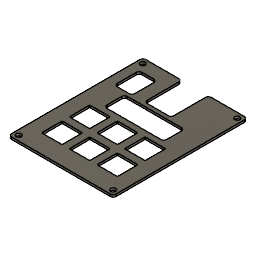
JONAHS LID (Autodesk Fusion 360 design; units mm, degrees)
part number: 2026-01-23-16-47-23-754
Autodesk Fusion 360 part; units mm, degrees
note: some values were not read from the file. Chosen so that the rebuilt part matches the saved one: which face or edge a step refers to; which pieces of a blend or face edit are solid. Set by a fixed rule: which sketch regions a step uses.
sketch "Sketch3" plane through (0, 0, 1.51) normal (0, 0, 1) x (-1, 0, 0)
  line L0 (-26.1938, 109.5375) -> (-88.1063, 109.5375)
  line L1 (-88.1063, 109.5375) -> (-88.1063, 27.245)
  line L2 (-88.1063, 27.245) -> (-26.1938, 27.245)
  line L3 (-26.1937, 27.245) -> (-26.1938, 109.5375)
  circle A0 centre (-33.02, 95.25) radius 0.85
  circle A1 centre (-34.29, 92.71) radius 0.75
  circle A2 centre (-38.1, 95.25) radius 2
  arc A3 (-43.3613, 96.0804) -> (-42.6772, 94.5646) centre (-43.18, 95.25) ccw
  arc A4 (-42.6772, 94.5646) -> (-43.3613, 96.0804) centre (-43.18, 95.25) ccw
  arc A5 (-40.9927, 90.8319) -> (-40.377, 89.4676) centre (-40.64, 90.17) ccw
  arc A6 (-40.377, 89.4676) -> (-40.9927, 90.8319) centre (-40.64, 90.17) ccw
  line L4 (-45.8755, 103.7524) -> (-46.5158, 103.0702)
  line L5 (-46.5158, 103.0702) -> (-46.5783, 103.1039)
  line L6 (-46.5783, 103.1039) -> (-46.8305, 103.1722)
  line L7 (-46.8305, 103.1722) -> (-48.4195, 103.1722)
  line L8 (-48.4195, 103.1722) -> (-48.6135, 103.1355)
  line L9 (-48.6135, 103.1355) -> (-48.6717, 103.1039)
  line L10 (-48.6717, 103.1039) -> (-49.403, 103.6875)
  line L11 (-49.403, 103.6875) -> (-49.3745, 103.7524)
  line L12 (-49.3745, 103.7524) -> (-49.325, 103.9693)
  line L13 (-49.325, 103.9693) -> (-49.325, 105.375)
  line L14 (-49.325, 105.375) -> (-49.3515, 105.5406)
  line L15 (-49.3515, 105.5406) -> (-49.3745, 105.5919)
  line L16 (-49.3745, 105.5919) -> (-48.7342, 106.2741)
  line L17 (-48.7342, 106.2741) -> (-48.6717, 106.2405)
  line L18 (-48.6717, 106.2405) -> (-48.4195, 106.1722)
  line L19 (-48.4195, 106.1722) -> (-46.8305, 106.1722)
  line L20 (-46.8305, 106.1722) -> (-46.6365, 106.2088)
  line L21 (-46.6365, 106.2088) -> (-46.5783, 106.2405)
  line L22 (-46.5783, 106.2405) -> (-45.847, 105.6568)
  line L23 (-45.847, 105.6568) -> (-45.8755, 105.5919)
  line L24 (-45.8755, 105.5919) -> (-45.925, 105.375)
  line L25 (-45.925, 105.375) -> (-45.925, 103.9693)
  line L26 (-45.925, 103.9693) -> (-45.8985, 103.8037)
  line L27 (-45.8985, 103.8037) -> (-45.8755, 103.7524)
  circle A7 centre (-52.07, 95.25) radius 0.85
  circle A8 centre (-53.34, 92.71) radius 0.75
  circle A9 centre (-57.15, 95.25) radius 2
  circle A10 centre (-33.02, 76.2) radius 0.85
  circle A11 centre (-34.29, 73.66) radius 0.75
  circle A12 centre (-38.1, 76.2) radius 2
  circle A13 centre (-43.18, 76.2) radius 0.85
  circle A14 centre (-40.64, 71.12) radius 0.75
  line L28 (-45.8105, 84.7036) -> (-46.4508, 84.0214)
  line L29 (-46.4508, 84.0214) -> (-46.5133, 84.0551)
  line L30 (-46.5133, 84.0551) -> (-46.7655, 84.1234)
  line L31 (-46.7655, 84.1234) -> (-48.3545, 84.1234)
  line L32 (-48.3545, 84.1234) -> (-48.5485, 84.0867)
  line L33 (-48.5485, 84.0867) -> (-48.6067, 84.0551)
  line L34 (-48.6067, 84.0551) -> (-49.338, 84.6387)
  line L35 (-49.338, 84.6387) -> (-49.3095, 84.7036)
  line L36 (-49.3095, 84.7036) -> (-49.26, 84.9205)
  line L37 (-49.26, 84.9205) -> (-49.26, 86.3262)
  line L38 (-49.26, 86.3262) -> (-49.2865, 86.4918)
  line L39 (-49.2865, 86.4918) -> (-49.3095, 86.5431)
  line L40 (-49.3095, 86.5431) -> (-48.6692, 87.2253)
  line L41 (-48.6692, 87.2253) -> (-48.6067, 87.1917)
  line L42 (-48.6067, 87.1917) -> (-48.3545, 87.1234)
  line L43 (-48.3545, 87.1234) -> (-46.7655, 87.1234)
  line L44 (-46.7655, 87.1234) -> (-46.5715, 87.16)
  line L45 (-46.5715, 87.16) -> (-46.5133, 87.1917)
  line L46 (-46.5133, 87.1917) -> (-45.782, 86.608)
  line L47 (-45.782, 86.608) -> (-45.8105, 86.5431)
  line L48 (-45.8105, 86.5431) -> (-45.86, 86.3262)
  line L49 (-45.86, 86.3262) -> (-45.86, 84.9205)
  line L50 (-45.86, 84.9205) -> (-45.8335, 84.7549)
  line L51 (-45.8335, 84.7549) -> (-45.8105, 84.7036)
  circle A15 centre (-52.07, 76.2) radius 0.85
  circle A16 centre (-53.34, 73.66) radius 0.75
  arc A17 (-59.1453, 76.3366) -> (-57.5161, 74.2338) centre (-57.15, 76.2) ccw
  arc A18 (-57.5161, 74.2338) -> (-59.1453, 76.3366) centre (-57.15, 76.2) ccw
  line L52 (-64.9255, 103.7524) -> (-65.5658, 103.0702)
  line L53 (-65.5658, 103.0702) -> (-65.6283, 103.1039)
  line L54 (-65.6283, 103.1039) -> (-65.8805, 103.1722)
  line L55 (-65.8805, 103.1722) -> (-67.4695, 103.1722)
  line L56 (-67.4695, 103.1722) -> (-67.6635, 103.1355)
  line L57 (-67.6635, 103.1355) -> (-67.7217, 103.1039)
  line L58 (-67.7217, 103.1039) -> (-68.453, 103.6875)
  line L59 (-68.453, 103.6875) -> (-68.4245, 103.7524)
  line L60 (-68.4245, 103.7524) -> (-68.375, 103.9693)
  line L61 (-68.375, 103.9693) -> (-68.375, 105.375)
  line L62 (-68.375, 105.375) -> (-68.4015, 105.5406)
  line L63 (-68.4015, 105.5406) -> (-68.4245, 105.5919)
  line L64 (-68.4245, 105.5919) -> (-67.7842, 106.2741)
  line L65 (-67.7842, 106.2741) -> (-67.7217, 106.2405)
  line L66 (-67.7217, 106.2405) -> (-67.4695, 106.1722)
  line L67 (-67.4695, 106.1722) -> (-65.8805, 106.1722)
  line L68 (-65.8805, 106.1722) -> (-65.6865, 106.2088)
  line L69 (-65.6865, 106.2088) -> (-65.6283, 106.2405)
  line L70 (-65.6283, 106.2405) -> (-64.897, 105.6568)
  line L71 (-64.897, 105.6568) -> (-64.9255, 105.5919)
  line L72 (-64.9255, 105.5919) -> (-64.975, 105.375)
  line L73 (-64.975, 105.375) -> (-64.975, 103.9693)
  line L74 (-64.975, 103.9693) -> (-64.9485, 103.8037)
  line L75 (-64.9485, 103.8037) -> (-64.9255, 103.7524)
  circle A19 centre (-62.23, 95.25) radius 0.85
  circle A20 centre (-59.69, 90.17) radius 0.75
  circle A21 centre (-71.12, 95.25) radius 0.85
  circle A22 centre (-72.39, 92.71) radius 0.75
  circle A23 centre (-76.2, 95.25) radius 2
  circle A24 centre (-81.28, 95.25) radius 0.85
  circle A25 centre (-78.74, 90.17) radius 0.75
  line L76 (-64.4728, 84.7212) -> (-65.1131, 84.039)
  line L77 (-65.1131, 84.039) -> (-65.1756, 84.0727)
  line L78 (-65.1756, 84.0727) -> (-65.4278, 84.141)
  line L79 (-65.4278, 84.141) -> (-67.0168, 84.141)
  line L80 (-67.0168, 84.141) -> (-67.2108, 84.1043)
  line L81 (-67.2108, 84.1043) -> (-67.269, 84.0727)
  line L82 (-67.269, 84.0727) -> (-68.0003, 84.6563)
  line L83 (-68.0003, 84.6563) -> (-67.9718, 84.7212)
  line L84 (-67.9718, 84.7212) -> (-67.9223, 84.9381)
  line L85 (-67.9223, 84.9381) -> (-67.9223, 86.3438)
  line L86 (-67.9223, 86.3438) -> (-67.9488, 86.5094)
  line L87 (-67.9488, 86.5094) -> (-67.9718, 86.5607)
  line L88 (-67.9718, 86.5607) -> (-67.3315, 87.2429)
  line L89 (-67.3315, 87.2429) -> (-67.269, 87.2093)
  line L90 (-67.269, 87.2093) -> (-67.0168, 87.141)
  line L91 (-67.0168, 87.141) -> (-65.4278, 87.141)
  line L92 (-65.4278, 87.141) -> (-65.2338, 87.1776)
  line L93 (-65.2338, 87.1776) -> (-65.1756, 87.2093)
  line L94 (-65.1756, 87.2093) -> (-64.4443, 86.6256)
  line L95 (-64.4443, 86.6256) -> (-64.4728, 86.5607)
  line L96 (-64.4728, 86.5607) -> (-64.5223, 86.3438)
  line L97 (-64.5223, 86.3438) -> (-64.5223, 84.9381)
  line L98 (-64.5223, 84.9381) -> (-64.4958, 84.7725)
  line L99 (-64.4958, 84.7725) -> (-64.4728, 84.7212)
  circle A26 centre (-68.95, 78.7) radius 0.5
  circle A27 centre (-62.23, 76.2) radius 0.85
  circle A28 centre (-59.69, 71.12) radius 0.75
  circle A29 centre (-68.95, 76.2) radius 0.5
  circle A30 centre (-68.95, 73.7) radius 0.5
  arc A31 (-77.1, 82.55) -> (-77.1, 81.05) centre (-77.1, 81.8) ccw
  line L100 (-77.1, 82.55) -> (-75.8, 82.55)
  arc A32 (-75.8, 81.05) -> (-75.8, 82.55) centre (-75.8, 81.8) ccw
  line L101 (-75.8, 81.05) -> (-77.1, 81.05)
  circle A33 centre (-83.45, 78.7) radius 0.5
  arc A34 (-77.1, 71.35) -> (-77.1, 69.85) centre (-77.1, 70.6) ccw
  line L102 (-77.1, 71.35) -> (-75.8, 71.35)
  arc A35 (-75.8, 69.85) -> (-75.8, 71.35) centre (-75.8, 70.6) ccw
  line L103 (-75.8, 69.85) -> (-77.1, 69.85)
  circle A36 centre (-83.45, 73.7) radius 0.5
  circle A37 centre (-40.4813, 61.9125) radius 0.5
  circle A38 centre (-40.4813, 59.3725) radius 0.5
  line L104 (-31.588, 56.1274) -> (-32.2283, 55.4452)
  line L105 (-32.2283, 55.4452) -> (-32.2908, 55.4789)
  line L106 (-32.2908, 55.4789) -> (-32.543, 55.5472)
  line L107 (-32.543, 55.5472) -> (-34.132, 55.5472)
  line L108 (-34.132, 55.5472) -> (-34.326, 55.5105)
  line L109 (-34.326, 55.5105) -> (-34.3842, 55.4789)
  line L110 (-34.3842, 55.4789) -> (-35.1155, 56.0625)
  line L111 (-35.1155, 56.0625) -> (-35.087, 56.1274)
  line L112 (-35.087, 56.1274) -> (-35.0375, 56.3443)
  line L113 (-35.0375, 56.3443) -> (-35.0375, 57.75)
  line L114 (-35.0375, 57.75) -> (-35.064, 57.9156)
  line L115 (-35.064, 57.9156) -> (-35.087, 57.9669)
  line L116 (-35.087, 57.9669) -> (-34.4467, 58.6491)
  line L117 (-34.4467, 58.6491) -> (-34.3842, 58.6155)
  line L118 (-34.3842, 58.6155) -> (-34.132, 58.5472)
  line L119 (-34.132, 58.5472) -> (-32.543, 58.5472)
  line L120 (-32.543, 58.5472) -> (-32.349, 58.5838)
  line L121 (-32.349, 58.5838) -> (-32.2908, 58.6155)
  line L122 (-32.2908, 58.6155) -> (-31.5595, 58.0318)
  line L123 (-31.5595, 58.0318) -> (-31.588, 57.9669)
  line L124 (-31.588, 57.9669) -> (-31.6375, 57.75)
  line L125 (-31.6375, 57.75) -> (-31.6375, 56.3443)
  line L126 (-31.6375, 56.3443) -> (-31.611, 56.1787)
  line L127 (-31.611, 56.1787) -> (-31.588, 56.1274)
  arc A39 (-40.8929, 57.1164) -> (-40.3451, 56.3514) centre (-40.4813, 56.8325) ccw
  arc A40 (-40.3451, 56.3514) -> (-40.8929, 57.1164) centre (-40.4813, 56.8325) ccw
  circle A41 centre (-40.4813, 54.2925) radius 0.5
  line L128 (-45.8755, 65.6524) -> (-46.5158, 64.9702)
  line L129 (-46.5158, 64.9702) -> (-46.5783, 65.0039)
  line L130 (-46.5783, 65.0039) -> (-46.8305, 65.0722)
  line L131 (-46.8305, 65.0722) -> (-48.4195, 65.0722)
  line L132 (-48.4195, 65.0722) -> (-48.6135, 65.0355)
  line L133 (-48.6135, 65.0355) -> (-48.6717, 65.0039)
  line L134 (-48.6717, 65.0039) -> (-49.403, 65.5875)
  line L135 (-49.403, 65.5875) -> (-49.3745, 65.6524)
  line L136 (-49.3745, 65.6524) -> (-49.325, 65.8693)
  line L137 (-49.325, 65.8693) -> (-49.325, 67.275)
  line L138 (-49.325, 67.275) -> (-49.3515, 67.4406)
  line L139 (-49.3515, 67.4406) -> (-49.3745, 67.4919)
  line L140 (-49.3745, 67.4919) -> (-48.7342, 68.1741)
  line L141 (-48.7342, 68.1741) -> (-48.6717, 68.1405)
  line L142 (-48.6717, 68.1405) -> (-48.4195, 68.0722)
  line L143 (-48.4195, 68.0722) -> (-46.8305, 68.0722)
  line L144 (-46.8305, 68.0722) -> (-46.6365, 68.1088)
  line L145 (-46.6365, 68.1088) -> (-46.5783, 68.1405)
  line L146 (-46.5783, 68.1405) -> (-45.847, 67.5568)
  line L147 (-45.847, 67.5568) -> (-45.8755, 67.4919)
  line L148 (-45.8755, 67.4919) -> (-45.925, 67.275)
  line L149 (-45.925, 67.275) -> (-45.925, 65.8693)
  line L150 (-45.925, 65.8693) -> (-45.8985, 65.7037)
  line L151 (-45.8985, 65.7037) -> (-45.8755, 65.6524)
  line L152 (-55.6192, 57.8615) -> (-56.2595, 57.1793)
  line L153 (-56.2595, 57.1793) -> (-56.322, 57.213)
  line L154 (-56.322, 57.213) -> (-56.5742, 57.2813)
  line L155 (-56.5742, 57.2813) -> (-58.1632, 57.2813)
  line L156 (-58.1632, 57.2813) -> (-58.3572, 57.2446)
  line L157 (-58.3572, 57.2446) -> (-58.4154, 57.213)
  line L158 (-58.4154, 57.213) -> (-59.1467, 57.7966)
  line L159 (-59.1467, 57.7966) -> (-59.1182, 57.8615)
  line L160 (-59.1182, 57.8615) -> (-59.0687, 58.0784)
  line L161 (-59.0687, 58.0784) -> (-59.0687, 59.4841)
  line L162 (-59.0687, 59.4841) -> (-59.0952, 59.6497)
  line L163 (-59.0952, 59.6497) -> (-59.1182, 59.701)
  line L164 (-59.1182, 59.701) -> (-58.4779, 60.3832)
  line L165 (-58.4779, 60.3832) -> (-58.4154, 60.3496)
  line L166 (-58.4154, 60.3496) -> (-58.1632, 60.2813)
  line L167 (-58.1632, 60.2813) -> (-56.5742, 60.2813)
  line L168 (-56.5742, 60.2813) -> (-56.3802, 60.3179)
  line L169 (-56.3802, 60.3179) -> (-56.322, 60.3496)
  line L170 (-56.322, 60.3496) -> (-55.5907, 59.7659)
  line L171 (-55.5907, 59.7659) -> (-55.6192, 59.701)
  line L172 (-55.6192, 59.701) -> (-55.6687, 59.4841)
  line L173 (-55.6687, 59.4841) -> (-55.6687, 58.0784)
  line L174 (-55.6687, 58.0784) -> (-55.6422, 57.9128)
  line L175 (-55.6422, 57.9128) -> (-55.6192, 57.8615)
  line L176 (-43.4606, 36.3505) -> (-43.8063, 36.3152)
  line L177 (-43.8063, 36.3152) -> (-43.9369, 36.3706)
  line L178 (-43.9369, 36.3706) -> (-44.1428, 36.9908)
  line L179 (-44.1428, 36.9908) -> (-44.1092, 37.0533)
  line L180 (-44.1092, 37.0533) -> (-44.0409, 37.3055)
  line L181 (-44.0409, 37.3055) -> (-44.0409, 38.8945)
  line L182 (-44.0409, 38.8945) -> (-44.0775, 39.0885)
  line L183 (-44.0775, 39.0885) -> (-44.1092, 39.1467)
  line L184 (-44.1092, 39.1467) -> (-43.5255, 39.878)
  line L185 (-43.5255, 39.878) -> (-43.4606, 39.8495)
  line L186 (-43.4606, 39.8495) -> (-43.2437, 39.8)
  line L187 (-43.2437, 39.8) -> (-41.838, 39.8)
  line L188 (-41.838, 39.8) -> (-41.6724, 39.8265)
  line L189 (-41.6724, 39.8265) -> (-41.6211, 39.8495)
  line L190 (-41.6211, 39.8495) -> (-40.9389, 39.2092)
  line L191 (-40.9389, 39.2092) -> (-40.9726, 39.1467)
  line L192 (-40.9726, 39.1467) -> (-41.0409, 38.8945)
  line L193 (-41.0409, 38.8945) -> (-41.0409, 37.3055)
  line L194 (-41.0409, 37.3055) -> (-41.0042, 37.1115)
  line L195 (-41.0042, 37.1115) -> (-40.9726, 37.0533)
  line L196 (-40.9726, 37.0533) -> (-41.5562, 36.322)
  line L197 (-41.5562, 36.322) -> (-41.6211, 36.3505)
  line L198 (-41.6211, 36.3505) -> (-41.838, 36.4)
  line L199 (-41.838, 36.4) -> (-43.2437, 36.4)
  line L200 (-43.2437, 36.4) -> (-43.4093, 36.3735)
  line L201 (-43.4093, 36.3735) -> (-43.4606, 36.3505)
  circle A42 centre (-49.525, 45.4025) radius 0.5
  circle A43 centre (-49.525, 42.8625) radius 0.5
  circle A44 centre (-49.525, 40.3225) radius 0.5
  circle A45 centre (-49.525, 37.7825) radius 0.5
  arc A46 (-50.0119, 35.3562) -> (-49.2555, 34.8214) centre (-49.525, 35.2425) ccw
  arc A47 (-49.2555, 34.8214) -> (-50.0119, 35.3562) centre (-49.525, 35.2425) ccw
  circle A48 centre (-49.525, 32.7025) radius 0.5
  circle A49 centre (-49.525, 30.1625) radius 0.5
  line L202 (-64.9255, 65.6524) -> (-65.5658, 64.9702)
  line L203 (-65.5658, 64.9702) -> (-65.6283, 65.0039)
  line L204 (-65.6283, 65.0039) -> (-65.8805, 65.0722)
  line L205 (-65.8805, 65.0722) -> (-67.4695, 65.0722)
  line L206 (-67.4695, 65.0722) -> (-67.6635, 65.0355)
  line L207 (-67.6635, 65.0355) -> (-67.7217, 65.0039)
  line L208 (-67.7217, 65.0039) -> (-68.453, 65.5875)
  line L209 (-68.453, 65.5875) -> (-68.4245, 65.6524)
  line L210 (-68.4245, 65.6524) -> (-68.375, 65.8693)
  line L211 (-68.375, 65.8693) -> (-68.375, 67.275)
  line L212 (-68.375, 67.275) -> (-68.4015, 67.4406)
  line L213 (-68.4015, 67.4406) -> (-68.4245, 67.4919)
  line L214 (-68.4245, 67.4919) -> (-67.7842, 68.1741)
  line L215 (-67.7842, 68.1741) -> (-67.7217, 68.1405)
  line L216 (-67.7217, 68.1405) -> (-67.4695, 68.0722)
  line L217 (-67.4695, 68.0722) -> (-65.8805, 68.0722)
  line L218 (-65.8805, 68.0722) -> (-65.6865, 68.1088)
  line L219 (-65.6865, 68.1088) -> (-65.6283, 68.1405)
  line L220 (-65.6283, 68.1405) -> (-64.897, 67.5568)
  line L221 (-64.897, 67.5568) -> (-64.9255, 67.4919)
  line L222 (-64.9255, 67.4919) -> (-64.975, 67.275)
  line L223 (-64.975, 67.275) -> (-64.975, 65.8693)
  line L224 (-64.975, 65.8693) -> (-64.9485, 65.7037)
  line L225 (-64.9485, 65.7037) -> (-64.9255, 65.6524)
  line L226 (-78.9942, 56.9802) -> (-79.6345, 56.298)
  line L227 (-79.6345, 56.298) -> (-79.697, 56.3317)
  line L228 (-79.697, 56.3317) -> (-79.9492, 56.4)
  line L229 (-79.9492, 56.4) -> (-81.5382, 56.4)
  line L230 (-81.5382, 56.4) -> (-81.7322, 56.3633)
  line L231 (-81.7322, 56.3633) -> (-81.7904, 56.3317)
  line L232 (-81.7904, 56.3317) -> (-82.5217, 56.9153)
  line L233 (-82.5217, 56.9153) -> (-82.4932, 56.9802)
  line L234 (-82.4932, 56.9802) -> (-82.4437, 57.1971)
  line L235 (-82.4437, 57.1971) -> (-82.4437, 58.6028)
  line L236 (-82.4437, 58.6028) -> (-82.4702, 58.7684)
  line L237 (-82.4702, 58.7684) -> (-82.4932, 58.8197)
  line L238 (-82.4932, 58.8197) -> (-81.8529, 59.5019)
  line L239 (-81.8529, 59.5019) -> (-81.7904, 59.4683)
  line L240 (-81.7904, 59.4683) -> (-81.5382, 59.4)
  line L241 (-81.5382, 59.4) -> (-79.9492, 59.4)
  line L242 (-79.9492, 59.4) -> (-79.7552, 59.4366)
  line L243 (-79.7552, 59.4366) -> (-79.697, 59.4683)
  line L244 (-79.697, 59.4683) -> (-78.9657, 58.8846)
  line L245 (-78.9657, 58.8846) -> (-78.9942, 58.8197)
  line L246 (-78.9942, 58.8197) -> (-79.0437, 58.6028)
  line L247 (-79.0437, 58.6028) -> (-79.0437, 57.1971)
  line L248 (-79.0437, 57.1971) -> (-79.0172, 57.0315)
  line L249 (-79.0172, 57.0315) -> (-78.9942, 56.9802)
  arc A50 (-64.9054, 45.8852) -> (-64.2764, 45.4405) centre (-64.775, 45.4025) ccw
  arc A51 (-64.2764, 45.4405) -> (-64.9054, 45.8852) centre (-64.775, 45.4025) ccw
  circle A52 centre (-64.775, 42.8625) radius 0.5
  circle A53 centre (-64.775, 40.3225) radius 0.5
  circle A54 centre (-64.775, 37.7825) radius 0.5
  circle A55 centre (-64.775, 35.2425) radius 0.5
  line L250 (-71.6073, 36.1317) -> (-71.9529, 36.0964)
  line L251 (-71.9529, 36.0964) -> (-72.0835, 36.1517)
  line L252 (-72.0835, 36.1517) -> (-72.2895, 36.772)
  line L253 (-72.2895, 36.772) -> (-72.2558, 36.8345)
  line L254 (-72.2558, 36.8345) -> (-72.1875, 37.0867)
  line L255 (-72.1875, 37.0867) -> (-72.1875, 38.6757)
  line L256 (-72.1875, 38.6757) -> (-72.2242, 38.8697)
  line L257 (-72.2242, 38.8697) -> (-72.2558, 38.9279)
  line L258 (-72.2558, 38.9279) -> (-71.6722, 39.6592)
  line L259 (-71.6722, 39.6592) -> (-71.6073, 39.6307)
  line L260 (-71.6073, 39.6307) -> (-71.3904, 39.5812)
  line L261 (-71.3904, 39.5812) -> (-69.9847, 39.5812)
  line L262 (-69.9847, 39.5812) -> (-69.8191, 39.6077)
  line L263 (-69.8191, 39.6077) -> (-69.7678, 39.6307)
  line L264 (-69.7678, 39.6307) -> (-69.0856, 38.9904)
  line L265 (-69.0856, 38.9904) -> (-69.1192, 38.9279)
  line L266 (-69.1192, 38.9279) -> (-69.1875, 38.6757)
  line L267 (-69.1875, 38.6757) -> (-69.1875, 37.0867)
  line L268 (-69.1875, 37.0867) -> (-69.1509, 36.8927)
  line L269 (-69.1509, 36.8927) -> (-69.1192, 36.8345)
  line L270 (-69.1192, 36.8345) -> (-69.7029, 36.1032)
  line L271 (-69.7029, 36.1032) -> (-69.7678, 36.1317)
  line L272 (-69.7678, 36.1317) -> (-69.9847, 36.1812)
  line L273 (-69.9847, 36.1812) -> (-71.3904, 36.1812)
  line L274 (-71.3904, 36.1812) -> (-71.556, 36.1547)
  line L275 (-71.556, 36.1547) -> (-71.6073, 36.1317)
  arc A56 (-65.2732, 32.7454) -> (-64.4428, 32.3288) centre (-64.775, 32.7025) ccw
  arc A57 (-64.4428, 32.3288) -> (-65.2732, 32.7454) centre (-64.775, 32.7025) ccw
  circle A58 centre (-64.775, 30.1625) radius 0.5
  line L276 (-28.5921, 104.14) -> (-85.598, 104.14)
  line L277 (-85.598, 104.14) -> (-85.598, 66.136)
  line L278 (-85.598, 66.136) -> (-28.5921, 66.136)
  line L279 (-28.5921, 66.136) -> (-28.5921, 104.14)
  line L280 (-50.6114, 68.6547) -> (-63.5786, 68.6547)
  arc A59 (-63.5786, 68.6547) -> (-64.0774, 69.1534) centre (-63.5786, 69.1534) cw
  line L281 (-64.0774, 69.1534) -> (-64.0774, 82.1206)
  arc A60 (-64.0774, 82.1206) -> (-63.5786, 82.6194) centre (-63.5786, 82.1206) cw
  line L282 (-63.5786, 82.6194) -> (-50.6114, 82.6194)
  arc A61 (-50.6114, 82.6194) -> (-50.1127, 82.1206) centre (-50.6114, 82.1206) cw
  line L283 (-50.1127, 82.1206) -> (-50.1127, 69.1534)
  arc A62 (-50.1127, 69.1534) -> (-50.6114, 68.6547) centre (-50.6114, 69.1534) cw
  line L284 (-50.6114, 87.6567) -> (-63.5786, 87.6567)
  arc A63 (-63.5786, 87.6567) -> (-64.0774, 88.1554) centre (-63.5786, 88.1554) cw
  line L285 (-64.0774, 88.1554) -> (-64.0774, 101.1226)
  arc A64 (-64.0774, 101.1226) -> (-63.5786, 101.6214) centre (-63.5786, 101.1226) cw
  line L286 (-63.5786, 101.6214) -> (-50.6114, 101.6214)
  arc A65 (-50.6114, 101.6214) -> (-50.1127, 101.1226) centre (-50.6114, 101.1226) cw
  line L287 (-50.1127, 101.1226) -> (-50.1127, 88.1554)
  arc A66 (-50.1127, 88.1554) -> (-50.6114, 87.6567) centre (-50.6114, 88.1554) cw
  line L288 (-69.6134, 87.6567) -> (-82.5806, 87.6567)
  arc A67 (-82.5806, 87.6567) -> (-83.0794, 88.1554) centre (-82.5806, 88.1554) cw
  line L289 (-83.0794, 88.1554) -> (-83.0794, 101.1226)
  arc A68 (-83.0794, 101.1226) -> (-82.5806, 101.6214) centre (-82.5806, 101.1226) cw
  line L290 (-82.5806, 101.6214) -> (-69.6134, 101.6214)
  arc A69 (-69.6134, 101.6214) -> (-69.1147, 101.1226) centre (-69.6134, 101.1226) cw
  line L291 (-69.1147, 101.1226) -> (-69.1147, 88.1554)
  arc A70 (-69.1147, 88.1554) -> (-69.6134, 87.6567) centre (-69.6134, 88.1554) cw
  line L292 (-31.6094, 68.6547) -> (-44.5767, 68.6547)
  arc A71 (-44.5767, 68.6547) -> (-45.0754, 69.1534) centre (-44.5767, 69.1534) cw
  line L293 (-45.0754, 69.1534) -> (-45.0754, 82.1206)
  arc A72 (-45.0754, 82.1206) -> (-44.5767, 82.6194) centre (-44.5767, 82.1206) cw
  line L294 (-44.5767, 82.6194) -> (-31.6094, 82.6194)
  arc A73 (-31.6094, 82.6194) -> (-31.1107, 82.1206) centre (-31.6094, 82.1206) cw
  line L295 (-31.1107, 82.1206) -> (-31.1107, 69.1534)
  arc A74 (-31.1107, 69.1534) -> (-31.6094, 68.6547) centre (-31.6094, 69.1534) cw
  line L296 (-31.6094, 87.6567) -> (-44.5767, 87.6567)
  arc A75 (-44.5767, 87.6567) -> (-45.0754, 88.1554) centre (-44.5767, 88.1554) cw
  line L297 (-45.0754, 88.1554) -> (-45.0754, 101.1226)
  arc A76 (-45.0754, 101.1226) -> (-44.5767, 101.6214) centre (-44.5767, 101.1226) cw
  line L298 (-44.5767, 101.6214) -> (-31.6094, 101.6214)
  arc A77 (-31.6094, 101.6214) -> (-31.1107, 101.1226) centre (-31.6094, 101.1226) cw
  line L299 (-31.1107, 101.1226) -> (-31.1107, 88.1554)
  arc A78 (-31.1107, 88.1554) -> (-31.6094, 87.6567) centre (-31.6094, 88.1554) cw
  line L300 (-93.1063, 114.5375) -> (-93.1063, 22.245)
  line L301 (-93.1063, 22.245) -> (-21.1938, 22.245)
  line L302 (-21.1937, 22.245) -> (-21.1938, 114.5375)
  line L303 (-21.1938, 114.5375) -> (-93.1062, 114.5375)
  circle A79 centre (-24.6938, 111.0375) radius 1.72
  circle A80 centre (-24.6937, 25.745) radius 1.72
  circle A81 centre (-89.6063, 25.745) radius 1.72
  circle A82 centre (-89.6063, 111.0375) radius 1.72
  line L304 (-69.1147, 82.6194) -> (-69.1147, 68.6194)
  line L305 (-69.1147, 68.6194) -> (-83.1147, 68.6194)
  line L306 (-83.1147, 68.6194) -> (-83.1147, 82.6194)
  line L307 (-83.1147, 82.6194) -> (-69.1147, 82.6194)
  line L308 (-29.6997, 33.245) -> (-29.6997, 46.245)
  line L309 (-29.6997, 33.245) -> (-37.6997, 33.245)
  line L310 (-37.6997, 33.245) -> (-37.6997, 46.245)
  line L311 (-37.6997, 46.245) -> (-29.6997, 46.245)
  line L312 (-39.6997, 48.245) -> (-27.6997, 48.245)
  line L313 (-27.6997, 31.245) -> (-27.6997, 48.245)
  line L314 (-27.6997, 31.245) -> (-39.6997, 31.245)
  line L315 (-39.6997, 31.245) -> (-39.6997, 48.245)
  line L316 (-65.275, 35.2425) -> (-66.275, 35.2425)
  line L317 (-49.025, 35.2425) -> (-48.025, 35.2425)
  line L318 (-64.775, 45.8852) -> (-64.775, 47.8852)
  line L319 (-49.525, 45.9025) -> (-49.525, 47.9025)
  line L320 (-49.525, 47.9025) -> (-48.025, 47.9025)
  line L321 (-48.025, 47.9025) -> (-48.025, 22.245)
  line L322 (-64.775, 47.8852) -> (-66.275, 47.8852)
  line L323 (-66.275, 47.8852) -> (-66.275, 22.245)
  line L324 (-64.775, 47.8852) -> (-49.525, 47.9025)
  line L325 (-38.4813, 54.2925) -> (-38.4813, 52.0925)
  line L326 (-38.4827, 61.9125) -> (-38.4827, 63.1125)
  line L327 (-38.4813, 52.0925) -> (-76.4813, 52.0925)
  line L328 (-76.4813, 52.0925) -> (-76.4813, 63.1125)
  line L329 (-76.4813, 63.1125) -> (-38.4827, 63.1125)
  line L330 (-38.4813, 52.0925) -> (-38.4827, 63.1125)
  line L331 (-38.4813, 50.5925) -> (-77.9813, 50.5925)
  line L332 (-77.9813, 50.5925) -> (-77.9813, 64.6125)
  line L333 (-77.9813, 64.6125) -> (-38.4827, 64.6125)
  line L334 (-38.4813, 50.5925) -> (-36.9813, 50.5927)
  line L335 (-36.9813, 50.5927) -> (-36.9813, 64.6125)
  line L336 (-36.9813, 64.6125) -> (-38.4827, 64.6125)
  dimension "d10" = 5
  dimension "d13" = 3.44
  dimension "d16" = 3.44
  dimension "d19" = 3.44
  dimension "d22" = 3.44
  dimension "d25" = 14
  dimension "d26" = 14
  dimension "d29" = 13
  dimension "d30" = 8
  dimension "d31" = 2
  dimension "d34" = 1
  dimension "d35" = 1
  dimension "d36" = 2
  dimension "d37" = 2
  dimension "d44" = 38
  dimension "d45" = -1.5
  dimension "d46" = 1.5
  constraint perpendicular L304 L305
  constraint perpendicular L305 L306
  constraint perpendicular L308 L309
  constraint perpendicular L309 L310
  constraint perpendicular L308 L311
  constraint coincident A55 L316.start
  constraint horizontal L316
  constraint coincident A47 L317.start
  constraint horizontal L317
  constraint vertical L318
  constraint coincident A42 L319.start
  constraint vertical L319
  constraint perpendicular L319 L320
  constraint coincident L301 L321.end
  constraint perpendicular L301 L321
  constraint perpendicular L318 L322
  constraint coincident L301 L323.end
  constraint perpendicular L301 L323
  constraint perpendicular L325 L327
  constraint perpendicular L167 L328
  constraint perpendicular L326 L329
  constraint perpendicular L330 L334
  constraint perpendicular L333 L335
  constraint perpendicular L335 L336
  measures "d13" diameter of A79
  measures "d16" diameter of A80
  measures "d19" diameter of A81
  measures "d22" diameter of A82
  measures "d25" distance of L304.start L304.end
  measures "d26" distance of L304.end L305.end
  measures "d29" distance of L308.start L308.end
  measures "d30" distance of L308.start L309.end
  measures "d34" distance of L316.start L316.end
  measures "d35" distance of L317.start L317.end
  measures "d36" distance of L318.start L318.end
  measures "d37" distance of L319.start L319.end
  measures "d44" distance of L325.end L327.end
  measures "d46" distance of L331.start L334.end
extrude "Extrude2" add sketch "Sketch3" along normal blind 1.5 contours L0 L1 L2 L3 L320 L321 L322 L323 L324 | L0 L1 L2 L3 L300 L301 L302 L303 L321 L323 | L4 L5 L6 L7 L8 L9 L10 L11 L12 L13 L25 L26 L27 L52 L53 L54 L55 L56 L57 L58 L59 L60 L61 L73 L74 L75 L137 L138 L139 L140 L141 L142 L143 L144 L145 L146 L147 L148 L149 L211 L212 L213 L214 L215 L216 L217 L218 L219 L220 L221 L222 L223 L276 L277 L278 L279 | L4 L5 L6 L7 L8 L9 L10 L11 L12 L13 L25 L26 L27 L276 | L13 L14 L15 L16 L17 L18 L19 L20 L21 L22 L23 L24 L25 L276 | L61 L62 L63 L64 L65 L66 L67 L68 L69 L70 L71 L72 L73 L276 | L52 L53 L54 L55 L56 L57 L58 L59 L60 L61 L73 L74 L75 L276 | L137 L138 L139 L140 L141 L142 L143 L144 L145 L146 L147 L148 L149 L278 | L128 L129 L130 L131 L132 L133 L134 L135 L136 L137 L149 L150 L151 L278 | L211 L212 L213 L214 L215 L216 L217 L218 L219 L220 L221 L222 L223 L278 | L202 L203 L204 L205 L206 L207 L208 L209 L210 L211 L223 L224 L225 L278 | L28 L29 L30 L31 L32 L33 L34 L35 L36 L37 L38 L39 L40 L41 L42 L43 L44 L45 L46 L47 L48 L49 L50 L51 | L76 L77 L78 L79 L80 L81 L82 L83 L84 L85 L86 L87 L88 L89 L90 L91 L92 L93 L94 L95 L96 L97 L98 L99 | A26 L304 | A29 L304 | A33 L306 | A30 L304 | A36 L306 | L104 L105 L106 L107 L108 L109 L110 L111 L112 L113 L114 L115 L116 L117 L118 L119 L120 L121 L122 L123 L124 L125 L126 L127 | L176 L177 L178 L179 L180 L181 L182 L183 L184 L185 L186 L187 L188 L189 L190 L191 L192 L193 L194 L195 L196 L197 L198 L199 L200 L201 | L226 L227 L228 L229 L230 L231 L232 L233 L234 L235 L236 L237 L238 L239 L240 L241 L242 L243 L244 L245 L246 L247 L248 L249 | L250 L251 L252 L253 L254 L255 L256 L257 L258 L259 L260 L261 L262 L263 L264 L265 L266 L267 L268 L269 L270 L271 L272 L273 L274 L275 picked at (-68.9064, 78.8284) picked at (-68.9064, 76.3284) picked at (-83.2922, 78.5695) picked at (-68.9064, 73.8284) picked at (-83.2922, 73.5695)
fillet "Fillet1" radius 2 4 edges at (93.1063, -114.5375, 2.26) (93.1063, -22.245, 2.26) (21.1937, -22.245, 2.26) (21.1938, -114.5375, 2.26)
fillet "Fillet2" radius 2 4 edges at (27.6997, -31.245, 2.26) (39.6997, -31.245, 2.26) (39.6997, -48.245, 2.26) (27.6997, -48.245, 2.26)
fillet "Fillet3" radius 2.0066 4 edges at (66.275, -47.8852, 2.26) (48.025, -47.9025, 2.26) (66.275, -22.245, 2.26) (48.025, -22.245, 2.26)
fillet "Fillet4" radius 2 4 edges at (77.9813, -64.6125, 2.26) (36.9813, -64.6125, 2.26) (77.9813, -50.5925, 2.26) (36.9813, -50.5927, 2.26)
